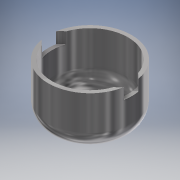
# Autodesk Inventor part: Hull
Saved by Autodesk Inventor 2016 (Build 200138000, 138)
## iProperties
Created: 2015-08-05
Part Number: Hull
Material: Generic
Document SubType Name: Modeling
Designer: 3DPrinterUser
Density: 1 g/cm^3
Appearance: Stainless - Brushed
Author: 3DPrinterUser
Autodesk Inventor part; units mm, degrees
ref_plane "YZ Plane" through (0, 0, 0) normal (1, 0, 0) x (0, 1, 0)
ref_plane "XY Plane" through (0, 0, 0) normal (0, 0, 1) x (1, 0, 0)
derived "Fixture.ipt"
sketch "Sketch1" plane through (0, 0, 0) normal (0, 1, 0) x (-1, 0, 0)
  line L0 (0, 0) -> (0, -76.5) construction
  line L1 (0, -76.5) -> (41.3, -76.5) construction
  line L2 (0, 0) -> (75.6, 0) construction
  line L3 (75.6, 0) -> (75.6, -45.99)
  line L4 (41.3, -76.5) -> (45.09, -76.5)
  arc A0 (45.09, -76.5) -> (75.6, -45.99) centre (45.09, -45.99) ccw
  line L5 (41.3, -76.5) -> (38.3, -76.5)
  line L6 (38.3, -76.5) -> (38.3, -79.5)
  line L7 (38.3, -79.5) -> (45.09, -79.5)
  arc A1 (45.09, -79.5) -> (78.6, -45.99) centre (45.09, -45.99) ccw
  line L8 (45.09, -76.5) -> (45.09, -79.5) construction
  line L9 (75.6, -45.99) -> (78.6, -45.99) construction
  line L10 (78.6, -45.99) -> (78.6, 0)
  line L11 (78.6, 0) -> (75.6, 0)
  line L12 (78.6, 0) -> (83.1, 0)
  line L13 (83.1, 0) -> (83.1, -45.99)
  arc A2 (45.09, -84) -> (83.1, -45.99) centre (45.09, -45.99) ccw
  line L14 (45.09, -84) -> (38.3, -84)
  line L15 (38.3, -84) -> (38.3, -79.5)
  dimension "d1" = 76.5
  dimension "d2" = 41.3
  dimension "d3" = 75.6
  dimension "d4" = 3
  dimension "d42" = 4.5
  constraints: 32 end point, 6 horizontal, 6 point on circle, 5 perpendicular, 5 vertical, 4 tangent, 3 centre point, 2 coincident, 1 point on line
  measures "d1" distance of L0.start L0.end
  measures "d2" distance of L0.end L1.end
  measures "d3" distance of L0.start L2.end
  measures "d4" distance of L1.end L5.end
  measures "d42" distance between parallel lines of L7 L14
revolve "Revolution1" add sketch "Sketch1" angle 360 about axis through (0, 0, 0) along (0, 0, -1)
sketch "Sketch3" plane through (0, 0, 0) normal (0, 0, 1) x (1, 0, 0)
  circle A0 centre (0, 0) radius 83.1 projected
  circle A1 centre (0, 0) radius 75.6 projected
derived "Transmission.ipt"
extrude "Extrusion1" add sketch "Sketch3" along normal blind 22.2
sketch "Sketch2" plane through (0, 0, 22.2) normal (0, 0, 1) x (1, 0, 0)
  circle A0 centre (58.45, 0) radius 25.45 construction
  circle A1 centre (0, 0) radius 75.6 construction
  line L0 (0, 0) -> (58.45, 0) construction
  circle A2 centre (58.45, 0) radius 27.45
  dimension "d6" = 58.45
  dimension "d7" = 50.9
  dimension "d11" = 2
  constraints: 2 centre point, 2 end point, 1 coincident, 1 horizontal
  measures "d6" distance of point (0, 0) L0.end
  measures "d7" diameter of A0
  measures "d11" radial gap between concentric circles of A0 A2
extrude "Extrusion2" cut sketch "Sketch2" against normal blind 22.2
mirror "Mirror3" about plane through (0, 0, 0) normal (1, 0, 0) of "Extrusion2"
sketch "Sketch4" plane through (0, 0, 22.2) normal (0, 0, 1) x (1, 0, 0)
  circle A0 centre (46.9447, -34.7427) radius 1.05 construction
  circle A1 centre (53.4135, -34.1066) radius 1.05 construction
  circle A2 centre (-46.9447, 34.7427) radius 1.05 construction
  circle A3 centre (-53.4135, 34.1066) radius 1.05 construction
  arc A4 (68.7665, 31.409) -> (72.8675, 20.1416) centre (71.0408, 25.8567) ccw construction
  arc A5 (68.7665, 31.409) -> (61.5843, 43.8491) centre (0, 0) ccw construction
  arc A6 (53.8769, 53.0343) -> (61.5843, 43.8491) centre (57.913, 48.5947) ccw construction
  arc A7 (53.8769, 53.0343) -> (42.873, 62.2677) centre (0, 0) ccw construction
  arc A8 (32.4889, 68.263) -> (42.873, 62.2677) centre (37.8, 65.4715) ccw construction
  arc A9 (32.4889, 68.263) -> (18.9906, 73.1759) centre (0, 0) ccw construction
  arc A10 (7.1823, 75.2581) -> (18.9906, 73.1759) centre (13.1278, 74.4515) ccw construction
  arc A11 (7.1823, 75.2581) -> (-7.1823, 75.2581) centre (0, 0) ccw construction
  arc A12 (-18.9906, 73.1759) -> (-7.1823, 75.2581) centre (-13.1278, 74.4515) ccw construction
  arc A13 (-18.9906, 73.1759) -> (-32.4889, 68.263) centre (0, 0) ccw construction
  arc A14 (-42.873, 62.2677) -> (-32.4889, 68.263) centre (-37.8, 65.4715) ccw construction
  arc A15 (-42.873, 62.2677) -> (-53.8769, 53.0343) centre (0, 0) ccw construction
  arc A16 (-61.5843, 43.8491) -> (-53.8769, 53.0343) centre (-57.913, 48.5947) ccw construction
  arc A17 (-61.5843, 43.8491) -> (-68.7665, 31.409) centre (0, 0) ccw construction
  arc A18 (-72.8675, 20.1416) -> (-68.7665, 31.409) centre (-71.0408, 25.8567) ccw construction
  arc A19 (-72.8675, 20.1416) -> (-72.8675, -20.1416) centre (0, 0) ccw construction
  arc A20 (-68.7665, -31.409) -> (-72.8675, -20.1416) centre (-71.0408, -25.8567) ccw construction
  arc A21 (-68.7665, -31.409) -> (-61.5843, -43.8491) centre (0, 0) ccw construction
  arc A22 (-53.8769, -53.0343) -> (-61.5843, -43.8491) centre (-57.913, -48.5947) ccw construction
  arc A23 (-53.8769, -53.0343) -> (-42.873, -62.2677) centre (0, 0) ccw construction
  arc A24 (-32.4889, -68.263) -> (-42.873, -62.2677) centre (-37.8, -65.4715) ccw construction
  arc A25 (-32.4889, -68.263) -> (-18.9906, -73.1759) centre (0, 0) ccw construction
  arc A26 (-7.1823, -75.2581) -> (-18.9906, -73.1759) centre (-13.1278, -74.4515) ccw construction
  arc A27 (-7.1823, -75.2581) -> (7.1823, -75.2581) centre (0, 0) ccw construction
  arc A28 (18.9906, -73.1759) -> (7.1823, -75.2581) centre (13.1278, -74.4515) ccw construction
  arc A29 (18.9906, -73.1759) -> (32.4889, -68.263) centre (0, 0) ccw construction
  arc A30 (42.873, -62.2677) -> (32.4889, -68.263) centre (37.8, -65.4715) ccw construction
  arc A31 (42.873, -62.2677) -> (53.8769, -53.0343) centre (0, 0) ccw construction
  arc A32 (61.5843, -43.8491) -> (53.8769, -53.0343) centre (57.913, -48.5947) ccw construction
  arc A33 (61.5843, -43.8491) -> (68.7665, -31.409) centre (0, 0) ccw construction
  arc A34 (72.8675, -20.1416) -> (68.7665, -31.409) centre (71.0408, -25.8567) ccw construction
  arc A35 (72.8675, -20.1416) -> (72.8675, 20.1416) centre (0, 0) ccw construction
  circle A36 centre (0, 0) radius 37.3 construction
  circle A37 centre (-58.45, 0) radius 11.5 construction
  circle A38 centre (58.45, 0) radius 11.5 construction
  circle A39 centre (-69.95, 11.5) radius 2.7 construction
  circle A40 centre (-46.95, -11.5) radius 2.7 construction
  circle A41 centre (69.95, 11.5) radius 2.7 construction
  circle A42 centre (46.95, -11.5) radius 2.7 construction
  circle A43 centre (69.95, -11.5) radius 2.7 construction
  circle A44 centre (46.95, 11.5) radius 2.7 construction
  circle A45 centre (-46.95, 11.5) radius 2.7 construction
  circle A46 centre (-69.95, -11.5) radius 2.7 construction
  circle A47 centre (60.2754, 34.8) radius 1.55 construction
  circle A48 centre (44.738, 53.3167) radius 1.55 construction
  circle A49 centre (16.1776, 44.4475) radius 1.55 construction
  circle A50 centre (0, 69.6) radius 1.55 construction
  circle A51 centre (-23.8046, 65.4026) radius 1.55 construction
  circle A52 centre (-30.4039, 36.2339) radius 1.55 construction
  circle A53 centre (-60.2754, 34.8) radius 1.55 construction
  circle A54 centre (60.2754, -34.8) radius 1.55 construction
  circle A55 centre (44.738, -53.3167) radius 1.55 construction
  circle A56 centre (23.8046, -65.4026) radius 1.55 construction
  circle A57 centre (-40.963, -23.65) radius 1.55 construction
  circle A58 centre (-30.4039, -36.2339) radius 1.55 construction
  circle A59 centre (-16.1776, -44.4475) radius 1.55 construction
  circle A60 centre (0, -47.3) radius 1.55 construction
  circle A61 centre (0, -69.6) radius 1.55 construction
  circle A62 centre (-23.8046, -65.4026) radius 1.55 construction
  circle A63 centre (-44.738, -53.3167) radius 1.55 construction
  circle A64 centre (-60.2754, -34.8) radius 1.55 construction
  circle A65 centre (16.1776, -44.4475) radius 1.55 construction
  circle A66 centre (30.4039, -36.2339) radius 1.55 construction
  circle A67 centre (40.963, -23.65) radius 1.55 construction
  circle A68 centre (-40.963, 23.65) radius 1.55 construction
  circle A69 centre (-44.738, 53.3167) radius 1.55 construction
  circle A70 centre (-16.1776, 44.4475) radius 1.55 construction
  circle A71 centre (0, 47.3) radius 1.55 construction
  circle A72 centre (23.8046, 65.4026) radius 1.55 construction
  circle A73 centre (30.4039, 36.2339) radius 1.55 construction
  circle A74 centre (40.963, 23.65) radius 1.55 construction
  arc A75 (7.1823, -75.2581) -> (18.9906, -73.1759) centre (0, 0) ccw
  arc A76 (18.9906, -73.1759) -> (7.1823, -75.2581) centre (13.1278, -74.4515) ccw
  constraints: 4 point on circle, 2 centre point, 2 coincident
sketch "Sketch12" plane through (0, 83.1, -22.995) normal (0, 1, 0) x (-1, 0, 0)
  line L0 (81.8521, 22.995) -> (81.8521, 45.195) projected
  line L1 (-81.8521, 45.195) -> (81.8521, 45.195) projected
  line L2 (-81.8521, 45.195) -> (-81.8521, 22.995) projected
  line L3 (-81.8521, 22.995) -> (-81.8521, 22.995) projected
  line L4 (-81.8521, 22.995) -> (-81.8521, 45.195) projected
  line L5 (81.8521, 45.195) -> (-81.8521, 45.195) projected
  line L6 (81.8521, 45.195) -> (81.8521, 22.995) projected
  line L7 (81.8521, 22.995) -> (81.8521, 22.995) projected
  line L8 (-83.1, -22.995) -> (83.1, -22.995) projected
  line L9 (81.8521, 22.995) -> (83.1, 22.995) projected
  line L10 (0, 22.995) -> (0, -22.995) construction
  point P0 (0, 0)
  constraints: 2 end point, 2 midpoint
sketch "Sketch11" plane through (0, 0, 0) normal (1, 0, 0) x (0, 1, 0)
  line L0 (75.7, -45.99) -> (75.7, 22.2) construction
  line L1 (75.7, -32.995) -> (80.7, -32.995)
  line L2 (80.7, -32.995) -> (80.7, -12.995)
  line L3 (80.7, -12.995) -> (75.7, -12.995)
  line L4 (75.7, -12.995) -> (75.7, -32.995)
  line L5 (80.7, -22.995) -> (75.7, -22.995) construction
  line L6 (0, -59.628) -> (0, 35.838) projected
  line L7 (75.7, -23.995) -> (83.1, -23.995) construction
  line L8 (75.7, -21.995) -> (83.1, -21.995) construction
  line L9 (75.7, -21.995) -> (83.1, -21.995) projected
  line L10 (80.7, -21.995) -> (80.7, -23.995)
  line L11 (75.7, -23.995) -> (83.1, -23.995) projected
  point P0 (0, 0)
  dimension "d44" = 5
  dimension "d45" = 20
  dimension "outer_hull_radius" = 83.1
  dimension "inner_hull_diameter" = 161.4
  constraints: 12 end point, 5 point on line, 3 midpoint, 2 parallel, 1 horizontal, 1 perpendicular
sketch "Sketch8" plane through (0, 0, -84) normal (0, 0, -1) x (-1, 0, 0)
  circle A0 centre (0, 0) radius 38.4
  circle A1 centre (0, 0) radius 58.8933
  circle A2 centre (0, -48.6467) radius 4.5
  line L0 (0, -44.1467) -> (0, -38.4) construction
  circle A3 centre (0, 0) radius 38.4 construction
  line L1 (0, -53.1467) -> (0, -58.8933) construction
  circle A4 centre (0, 0) radius 58.8933 construction
  line L2 (0, -38.4) -> (0, 0) construction
  dimension "d38" = 9
  constraints: 6 end point, 4 vertical alignment, 3 vertical, 2 line through centre, 2 point on circle, 1 centre point, 1 collinear, 8 other
  measures "d38" diameter of A2
equation "\"d1\" = fixture_height + stand_height"
equation "\"d2\" = 0.5 * pvc_radius + thickness"
equation "\"d3\" = 0.5 * outer_radius"
equation "\"d4\" = thickness"
equation "\"d42\" = 1.5 * thickness"
equation "\"d9\" = height_1 + 2 * transmission_gap"
equation "\"d6\" = stepper_center_distance"
equation "\"d7\" = transmission_diameter"
equation "\"d12\" = height_1 + 2 * transmission_gap"
equation "\"d38\" = 3 * thickness"
equation "\"led_distance\" = 31"
equation "\"fixture_height\" = 72"
equation "\"stand_height\" = 4.5"
equation "\"pvc_radius\" = 76.6"
equation "\"thickness\" = 3"
equation "\"outer_radius\" = 151.2"
equation "\"height_1\" = 21"
equation "\"transmission_gap\" = 0.6"
equation "\"transmission_diameter\" = 50.9"
equation "\"stepper_center_distance\" = 58.45"
body "Solid1"
